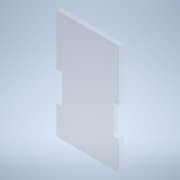
# Autodesk Inventor part: box_layout
Saved by Autodesk Inventor 2020 (Build 240168000, 168)
## iProperties
Created: 2019-10-22
Part Number: box_layout
Material: Polycarbonate, Clear
Document SubType Name: Modeling
Designer: Connor
Density: 1.2 g/cm^3
Appearance: Polycarbonate - Clear
Mass: 803.171 g
Surface Area: 1186.29 cm^2
Volume: 669.309 cm^3
Author: Connor
Autodesk Inventor part; units mm, degrees
ref_plane "YZ Plane" through (0, 0, 0) normal (1, 0, 0) x (0, 1, 0)
ref_plane "XZ Plane" through (0, 0, 0) normal (0, 1, 0) x (-1, 0, 0)
ref_plane "XY Plane" through (0, 0, 0) normal (0, 0, 1) x (1, 0, 0)
sketch "Sketch2" plane through (0, 0, 0) normal (0, 0, 1) x (1, 0, 0)
  line L0 (0, 311.15) -> (177.8, 311.15)
  line L1 (177.8, 0) -> (0, 0)
  line L2 (15.875, 165.4048) -> (0, 165.4048)
  line L3 (15.875, 165.4048) -> (15.875, 82.8548)
  line L4 (15.875, 82.8548) -> (0, 82.8548)
  line L5 (177.8, 165.4048) -> (161.925, 165.4048)
  line L6 (161.925, 165.4048) -> (161.925, 82.8548)
  line L7 (161.925, 82.8548) -> (177.8, 82.8548)
  line L8 (0, 0) -> (0, 82.8548)
  line L9 (0, 165.4048) -> (0, 311.15)
  line L10 (177.8, 311.15) -> (177.8, 165.4048)
  line L11 (177.8, 82.8548) -> (177.8, 0)
  dimension "d11" = 311.15
  dimension "d12" = 177.8
  dimension "d14" = 15.875
  dimension "d15" = 82.55
  dimension "d16" = 15.875
  dimension "d17" = 82.55
  constraints: 24 end point, 11 perpendicular, 3 vertical, 2 horizontal
  measures "d11" distance of L1.end L0.start
  measures "d12" distance of L0.start L0.end
  measures "d14" distance of L2.start L2.end
  measures "d15" distance of L2.start L3.end
  measures "d16" distance of L5.start L5.end
  measures "d17" distance of L5.end L6.end
extrude "Extrusion2" add sketch "Sketch2" along normal blind 12.7
body "Solid2"
